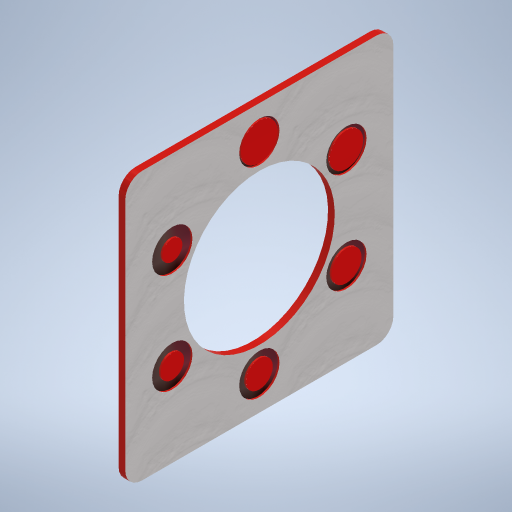
# Autodesk Inventor part: parte4
Saved by Autodesk Inventor 2024 (Build 280153000, 153)
## iProperties
Created: 2023-12-18
Part Number: parte4
Material: Generico
Document SubType Name: Modeling
Designer: cecca
Density: 1 g/cm^3
Appearance: Rosso arancio
Author: cecca
Autodesk Inventor part; units mm, degrees
ref_plane "YZ Plane" through (0, 0, 0) normal (1, 0, 0) x (0, 1, 0)
ref_plane "XZ Plane" through (0, 0, 0) normal (0, 1, 0) x (-1, 0, 0)
ref_plane "XY Plane" through (0, 0, 0) normal (0, 0, 1) x (1, 0, 0)
sketch "Schizzo1" plane through (0, 0, 0) normal (1, 0, 0) x (0, 1, 0)
  line L0 (-35, -40) -> (35, -40)
  line L1 (40, -35) -> (40, 35)
  line L2 (35, 40) -> (-35, 40)
  line L3 (-40, 35) -> (-40, -35)
  line L4 (-40, -40) -> (40, 40) construction
  line L5 (40, -40) -> (-40, 40) construction
  arc A0 (40, 35) -> (35, 40) centre (35, 35) ccw
  arc A1 (35, -40) -> (40, -35) centre (35, -35) ccw
  arc A2 (-35, 40) -> (-40, 35) centre (-35, 35) ccw
  arc A3 (-40, -35) -> (-35, -40) centre (-35, -35) ccw
  circle A4 centre (0, 0) radius 22.5
  dimension "d4" = 45
  constraints: 12 end point, 8 point on circle, 5 centre point, 2 midpoint, 2 parallel, 1 coincident, 1 horizontal, 1 perpendicular
  measures "d4" diameter of A4
extrude "Estrusione1" add sketch "Schizzo1" along normal mid plane 2
sketch "Schizzo2" plane through (1, 0, 0) normal (1, 0, 0) x (0, 0, -1)
  circle A0 centre (0, 0) radius 30
  circle A1 centre (0, 30) radius 6.0177
  circle A2 centre (-25.9808, 15) radius 6.0177
  circle A3 centre (-25.9808, -15) radius 6.0177
  circle A4 centre (0, -30) radius 6.0177
  circle A5 centre (25.9808, -15) radius 6.0177
  circle A6 centre (25.9808, 15) radius 6.0177
  circle A7 centre (-25.9808, 15) radius 5.5175
  circle A8 centre (-25.9808, 15) radius 5.0175
  circle A9 centre (-25.9808, 15) radius 4.5175
  circle A10 centre (-25.9808, 15) radius 4.0175
  circle A11 centre (-25.9808, 15) radius 3.5175
  circle A12 centre (0, -30) radius 6.0177
  circle A13 centre (-25.9808, -15) radius 3.5175
  circle A14 centre (-25.9808, -15) radius 4.0175
  circle A15 centre (-25.9808, -15) radius 4.5175
  circle A16 centre (-25.9808, -15) radius 5.0175
  circle A17 centre (-25.9808, -15) radius 5.5175
  circle A18 centre (25.9808, -15) radius 6.0177
  circle A19 centre (0, -30) radius 3.5175
  circle A20 centre (0, -30) radius 4.0175
  circle A21 centre (0, -30) radius 4.5175
  circle A22 centre (0, -30) radius 5.0175
  circle A23 centre (0, -30) radius 5.5175
  circle A24 centre (25.9808, 15) radius 6.0177
  circle A25 centre (25.9808, -15) radius 3.5175
  circle A26 centre (25.9808, -15) radius 4.0175
  circle A27 centre (25.9808, -15) radius 4.5175
  circle A28 centre (25.9808, -15) radius 5.0175
  circle A29 centre (25.9808, -15) radius 5.5175
  circle A30 centre (0, 30) radius 6.0177
  circle A31 centre (25.9808, 15) radius 3.5175
  circle A32 centre (25.9808, 15) radius 4.0175
  circle A33 centre (25.9808, 15) radius 4.5175
  circle A34 centre (25.9808, 15) radius 5.0175
  circle A35 centre (25.9808, 15) radius 5.5175
  circle A36 centre (-25.9808, 15) radius 6.0177
  circle A37 centre (0, 30) radius 3.5175
  circle A38 centre (0, 30) radius 4.0175
  circle A39 centre (0, 30) radius 4.5175
  circle A40 centre (0, 30) radius 5.0175
  circle A41 centre (0, 30) radius 5.5175
  circle A42 centre (-25.9808, 15) radius 3.0175
  dimension "d7" = 60
  dimension "d10" = 360
  dimension "d13" = 11.035
  dimension "d14" = 10.035
  dimension "d15" = 9.035
  dimension "d16" = 8.035
  dimension "d17" = 7.035
  dimension "d20" = 360
  dimension "d24" = 6.035
  constraints: 43 centre point, 20 coincident, 2 point on circle, 86 other
  measures "d7" diameter of A0
  measures "d13" diameter of A7
  measures "d14" diameter of A8
  measures "d15" diameter of A9
  measures "d16" diameter of A10
  measures "d17" diameter of A11
  measures "d24" diameter of A42
extrude "Estrusione2" cut sketch "Schizzo2" against normal blind 0.5 contours A6 A0 A35 | A0 A35 A6 | A5 A0 A29 | A0 A29 A5 | A35 A0 A34 | A0 A34 A35 | A29 A0 A28 | A0 A28 A29 | A1 A0 A41 | A0 A41 A1 | A28 A0 A27 | A0 A27 A28 | A4 A0 A23 | A0 A23 A4 | A23 A0 A22 | A0 A22 A23 | A2 A0 A7 | A0 A7 A2 | A22 A0 A21 | A0 A21 A22 | A3 A0 A17 | A0 A17 A3 | A7 A0 A8 | A0 A8 A7 | A21 A0 A20 | A0 A20 A21 | A17 A0 A16 | A0 A16 A17 | A8 A0 A9 | A0 A9 A8 | A16 A0 A15 | A0 A15 A16 | A9 A0 A10 | A0 A10 A9 | A15 A0 A14 | A0 A14 A15 | A10 A0 A11 | A0 A11 A10 | A14 A0 A13 | A0 A13 A14 | A11 A0 A42 | A0 A42 A11
